Autodesk Fusion 360 part; units mm, degrees
(part 2 of 5)
  spline S63 degree 5 poles (8.5628, 46.3914) (8.5526, 46.3783) (8.5324, 46.3521) (8.5021, 46.3128) (8.4619, 46.2602) (8.4119, 46.1945) (8.3623, 46.1286) (8.3129, 46.0625) (8.2639, 45.9964) (8.2152, 45.9301) (8.1668, 45.8637) (8.1187, 45.7971) (8.0709, 45.7305) (8.0235, 45.6637) (7.9764, 45.5967) (7.9296, 45.5297) (7.8831, 45.4625) (7.837, 45.3952) (7.7912, 45.3278) (7.7458, 45.2602) (7.7007, 45.1925) (7.6639, 45.1368) (7.6362, 45.0946) (7.6175, 45.0659) (7.6077, 45.0508) (7.6067, 45.0493) knots -1 -1 -1 -1 -1 -1 -0.985714 -0.971429 -0.957143 -0.942857 -0.928571 -0.914286 -0.9 -0.885714 -0.871429 -0.857143 -0.842857 -0.828571 -0.814286 -0.8 -0.785714 -0.771429 -0.757143 -0.742857 -0.728571 -0.714286 -0.712736 -0.712736 -0.712736 -0.712736 -0.712736 -0.712736
  line L43 (-7.433, 28.7473) -> (-9.4231, 36.4981)
  line L44 (-10.9838, 27.4883) -> (-13.9296, 34.9285)
  spline S64 degree 5 poles (-12.2983, -44.0007) (-12.2981, -44.0024) (-12.2956, -44.0202) (-12.2909, -44.0541) (-12.2838, -44.1041) (-12.2743, -44.1702) (-12.2623, -44.2506) (-12.2499, -44.3311) (-12.2372, -44.4116) (-12.2241, -44.4922) (-12.2107, -44.5727) (-12.1969, -44.6533) (-12.1828, -44.734) (-12.1683, -44.8146) (-12.1534, -44.8953) (-12.1383, -44.9759) (-12.1228, -45.0566) (-12.1069, -45.1374) (-12.0907, -45.2181) (-12.0742, -45.2989) (-12.0573, -45.3796) (-12.0401, -45.4604) (-12.0261, -45.525) (-12.0154, -45.5735) (-12.0083, -45.6059) (-12.0047, -45.622) knots 0.712736 0.712736 0.712736 0.712736 0.712736 0.712736 0.714286 0.728571 0.742857 0.757143 0.771429 0.785714 0.8 0.814286 0.828571 0.842857 0.857143 0.871429 0.885714 0.9 0.914286 0.928571 0.942857 0.957143 0.971429 0.985714 1 1 1 1 1 1
  arc A63 (-23.9559, 16.8474) -> (-24.9507, 15.2942) centre (0.7975, -0.1016) ccw
  line L45 (22.0846, 21.0374) -> (27.7612, 26.6745)
  line L46 (-21.6364, 19.8162) -> (-27.6188, 25.1276)
  arc A64 (-21.6364, 19.8162) -> (-22.8181, 18.3999) centre (0.7975, -0.1016) ccw
  arc A65 (-37.0211, 3.6065) -> (-37.1692, 1.488) centre (0.7975, -0.1016) ccw
  arc A66 (-9.1163, -46.2858) -> (-8.5628, -46.3914) centre (0, 0) ccw
  spline S65 degree 5 poles (-19.8308, -42.8044) (-19.8177, -42.7943) (-19.7916, -42.7739) (-19.7525, -42.7434) (-19.7005, -42.7025) (-19.6357, -42.6512) (-19.5713, -42.5997) (-19.5071, -42.5481) (-19.4431, -42.4962) (-19.3794, -42.4441) (-19.3161, -42.3918) (-19.2529, -42.3393) (-19.1901, -42.2866) (-19.1275, -42.2337) (-19.0652, -42.1806) (-19.0032, -42.1273) (-18.9415, -42.0738) (-18.8801, -42.02) (-18.819, -41.9661) (-18.7582, -41.912) (-18.6976, -41.8576) (-18.6481, -41.8128) (-18.6109, -41.7788) (-18.5856, -41.7557) (-18.5724, -41.7435) (-18.5711, -41.7423) knots -1 -1 -1 -1 -1 -1 -0.985714 -0.971429 -0.957143 -0.942857 -0.928571 -0.914286 -0.9 -0.885714 -0.871429 -0.857143 -0.842857 -0.828571 -0.814286 -0.8 -0.785714 -0.771429 -0.757143 -0.742857 -0.728571 -0.714286 -0.712736 -0.712736 -0.712736 -0.712736 -0.712736 -0.712736
  spline S66 degree 3 poles (-6.6866, -45.1951) (-6.7038, -45.1309) (-6.7334, -45.0708) (-6.8139, -44.9652) (-6.8641, -44.9207) (-6.9787, -44.8536) (-7.0421, -44.8316) (-7.1736, -44.813) (-7.2405, -44.8167) (-7.3692, -44.8494) (-7.4298, -44.8782) (-7.5318, -44.9539) (-7.5737, -44.9985) (-7.6067, -45.0493) knots 0 0 0 0 0.019923 0.019923 0.039846 0.039846 0.059769 0.059769 0.079691 0.079691 0.099614 0.099614 0.117812 0.117812 0.117812 0.117812
  line L47 (-18.9632, 22.4708) -> (-24.2327, 28.4902)
  line L48 (-29.0593, 2.8259) -> (-37.0211, 3.6065)
  arc A67 (-30.5568, 21.3671) -> (-31.7072, 19.582) centre (0.7975, -0.1016) ccw
  spline S67 degree 3 poles (9.5112, 44.686) (9.5244, 44.621) (9.5501, 44.5591) (9.6239, 44.4486) (9.6712, 44.4011) (9.7814, 44.3269) (9.8432, 44.301) (9.9732, 44.2742) (10.0403, 44.2736) (10.1708, 44.2982) (10.233, 44.3231) (10.3396, 44.3923) (10.3842, 44.4341) (10.4204, 44.4828) knots 0 0 0 0 0.019923 0.019923 0.039846 0.039846 0.059769 0.059769 0.079691 0.079691 0.099614 0.099614 0.117812 0.117812 0.117812 0.117812
  spline S68 degree 3 poles (12.2983, 44.0007) (12.3073, 43.9349) (12.3291, 43.8715) (12.3958, 43.7566) (12.4401, 43.7062) (12.5454, 43.6253) (12.6054, 43.5955) (12.7336, 43.5606) (12.8004, 43.5558) (12.9322, 43.5721) (12.9959, 43.5931) (13.1066, 43.6555) (13.1538, 43.6944) (13.1929, 43.7407) knots 0 0 0 0 0.019923 0.019923 0.039846 0.039846 0.059769 0.059769 0.079691 0.079691 0.099614 0.099614 0.117812 0.117812 0.117812 0.117812
  arc A68 (-25.885, 13.6113) -> (-26.6773, 11.9457) centre (0.7975, -0.1016) ccw
  spline S69 degree 3 poles (6.6866, 45.1951) (6.7038, 45.1309) (6.7334, 45.0708) (6.8139, 44.9652) (6.8641, 44.9207) (6.9787, 44.8536) (7.0421, 44.8316) (7.1736, 44.813) (7.2405, 44.8167) (7.3692, 44.8494) (7.4298, 44.8782) (7.5318, 44.9539) (7.5737, 44.9985) (7.6067, 45.0493) knots 0 0 0 0 0.019923 0.019923 0.039846 0.039846 0.059769 0.059769 0.079691 0.079691 0.099614 0.099614 0.117812 0.117812 0.117812 0.117812
  arc A69 (-12.0047, -45.622) -> (-11.4588, -45.7622) centre (0, 0) ccw
  line L49 (17.7796, 24.6291) -> (22.4832, 31.103)
  arc A70 (-34.9108, 12.8952) -> (-35.5811, 10.88) centre (0.7975, -0.1016) ccw
  line L50 (-24.9507, 15.2942) -> (-31.7072, 19.582)
  spline S70 degree 5 poles (-0.2818, 47.1742) (-0.2893, 47.1594) (-0.3043, 47.1299) (-0.3267, 47.0856) (-0.3563, 47.0264) (-0.3931, 46.9525) (-0.4295, 46.8784) (-0.4656, 46.8043) (-0.5013, 46.7302) (-0.5368, 46.6559) (-0.5719, 46.5816) (-0.6066, 46.5072) (-0.641, 46.4328) (-0.6751, 46.3583) (-0.7089, 46.2837) (-0.7423, 46.2091) (-0.7753, 46.1344) (-0.808, 46.0596) (-0.8404, 45.9848) (-0.8723, 45.9099) (-0.904, 45.835) (-0.9297, 45.7734) (-0.9489, 45.7267) (-0.9619, 45.695) (-0.9687, 45.6784) (-0.9694, 45.6768) knots -1 -1 -1 -1 -1 -1 -0.985714 -0.971429 -0.957143 -0.942857 -0.928571 -0.914286 -0.9 -0.885714 -0.871429 -0.857143 -0.842857 -0.828571 -0.814286 -0.8 -0.785714 -0.771429 -0.757143 -0.742857 -0.728571 -0.714286 -0.712736 -0.712736 -0.712736 -0.712736 -0.712736 -0.712736
  arc A71 (-36.2582, 8.3172) -> (-36.6706, 6.2339) centre (0.7975, -0.1016) ccw
  spline S71 degree 5 poles (19.8308, 42.8044) (19.8177, 42.7943) (19.7916, 42.7739) (19.7525, 42.7434) (19.7005, 42.7025) (19.6357, 42.6512) (19.5713, 42.5997) (19.5071, 42.5481) (19.4431, 42.4962) (19.3794, 42.4441) (19.3161, 42.3918) (19.2529, 42.3393) (19.1901, 42.2866) (19.1275, 42.2337) (19.0652, 42.1806) (19.0032, 42.1273) (18.9415, 42.0738) (18.8801, 42.02) (18.819, 41.9661) (18.7582, 41.912) (18.6976, 41.8576) (18.6481, 41.8128) (18.6109, 41.7788) (18.5856, 41.7557) (18.5724, 41.7435) (18.5711, 41.7423) knots -1 -1 -1 -1 -1 -1 -0.985714 -0.971429 -0.957143 -0.942857 -0.928571 -0.914286 -0.9 -0.885714 -0.871429 -0.857143 -0.842857 -0.828571 -0.814286 -0.8 -0.785714 -0.771429 -0.757143 -0.742857 -0.728571 -0.714286 -0.712736 -0.712736 -0.712736 -0.712736 -0.712736 -0.712736
  spline S72 degree 3 poles (0.9694, 45.6768) (0.9945, 45.6153) (1.0314, 45.5593) (1.1246, 45.4646) (1.1799, 45.4268) (1.3021, 45.3746) (1.3676, 45.3607) (1.5004, 45.3587) (1.5664, 45.3707) (1.69, 45.4194) (1.7465, 45.4555) (1.8382, 45.5434) (1.8742, 45.5929) (1.9006, 45.6475) knots 0 0 0 0 0.019923 0.019923 0.039846 0.039846 0.059769 0.059769 0.079691 0.079691 0.099614 0.099614 0.117812 0.117812 0.117812 0.117812
  spline S73 degree 3 poles (-3.8356, -45.5258) (-3.8568, -45.4628) (-3.8901, -45.4046) (-3.9771, -45.3043) (-4.03, -45.2631) (-4.1486, -45.2033) (-4.2132, -45.1853) (-4.3456, -45.175) (-4.4122, -45.1829) (-4.5386, -45.2236) (-4.5972, -45.2562) (-4.6943, -45.3381) (-4.7333, -45.3852) (-4.7631, -45.4381) knots 0 0 0 0 0.019923 0.019923 0.039846 0.039846 0.059769 0.059769 0.079691 0.079691 0.099614 0.099614 0.117812 0.117812 0.117812 0.117812
  line L51 (-29.1828, 0.9855) -> (-37.1692, 1.488)
  spline S74 degree 5 poles (-5.6329, -46.8375) (-5.6236, -46.8238) (-5.6051, -46.7964) (-5.5773, -46.7552) (-5.5405, -46.7003) (-5.4947, -46.6315) (-5.4493, -46.5626) (-5.4042, -46.4936) (-5.3595, -46.4245) (-5.315, -46.3553) (-5.2709, -46.286) (-5.2271, -46.2165) (-5.1836, -46.147) (-5.1404, -46.0774) (-5.0976, -46.0076) (-5.0551, -45.9377) (-5.013, -45.8678) (-4.9712, -45.7977) (-4.9297, -45.7275) (-4.8886, -45.6572) (-4.8478, -45.5869) (-4.8146, -45.5289) (-4.7896, -45.4851) (-4.7728, -45.4553) (-4.7639, -45.4396) (-4.7631, -45.4381) knots -1 -1 -1 -1 -1 -1 -0.985714 -0.971429 -0.957143 -0.942857 -0.928571 -0.914286 -0.9 -0.885714 -0.871429 -0.857143 -0.842857 -0.828571 -0.814286 -0.8 -0.785714 -0.771429 -0.757143 -0.742857 -0.728571 -0.714286 -0.712736 -0.712736 -0.712736 -0.712736 -0.712736 -0.712736
  spline S75 degree 3 poles (15.0368, 43.1416) (15.0417, 43.0754) (15.0595, 43.0107) (15.1189, 42.8919) (15.1599, 42.8389) (15.2599, 42.7515) (15.3179, 42.718) (15.4436, 42.6751) (15.5101, 42.6661) (15.6426, 42.6741) (15.7075, 42.6911) (15.8219, 42.7464) (15.8714, 42.7823) (15.9134, 42.826) knots 0 0 0 0 0.019923 0.019923 0.039846 0.039846 0.059769 0.059769 0.079691 0.079691 0.099614 0.099614 0.117812 0.117812 0.117812 0.117812
  spline S76 degree 3 poles (-15.0368, -43.1416) (-15.0417, -43.0754) (-15.0595, -43.0107) (-15.1189, -42.8919) (-15.1599, -42.8389) (-15.2599, -42.7515) (-15.3179, -42.718) (-15.4436, -42.6751) (-15.5101, -42.6661) (-15.6426, -42.6741) (-15.7075, -42.6911) (-15.8219, -42.7464) (-15.8714, -42.7823) (-15.9134, -42.826) knots 0 0 0 0 0.019923 0.019923 0.039846 0.039846 0.059769 0.059769 0.079691 0.079691 0.099614 0.099614 0.117812 0.117812 0.117812 0.117812
  spline S77 degree 3 poles (17.7161, 42.1123) (17.7168, 42.0459) (17.7305, 41.9803) (17.7822, 41.858) (17.8198, 41.8024) (17.9141, 41.7089) (17.97, 41.6718) (18.0927, 41.6211) (18.1585, 41.608) (18.2913, 41.6077) (18.3571, 41.6206) (18.4748, 41.6685) (18.5264, 41.7013) (18.5711, 41.7423) knots 0 0 0 0 0.019923 0.019923 0.039846 0.039846 0.059769 0.059769 0.079691 0.079691 0.099614 0.099614 0.117812 0.117812 0.117812 0.117812
  spline S78 degree 5 poles (-17.7161, -42.1123) (-17.716, -42.1141) (-17.7158, -42.1321) (-17.7154, -42.1663) (-17.7147, -42.2168) (-17.7135, -42.2835) (-17.7117, -42.3648) (-17.7095, -42.4462) (-17.707, -42.5277) (-17.7041, -42.6093) (-17.7008, -42.6909) (-17.6973, -42.7726) (-17.6933, -42.8543) (-17.6891, -42.9361) (-17.6845, -43.018) (-17.6795, -43.1) (-17.6743, -43.182) (-17.6686, -43.264) (-17.6627, -43.3462) (-17.6564, -43.4284) (-17.6498, -43.5106) (-17.6429, -43.5929) (-17.6371, -43.6588) (-17.6326, -43.7082) (-17.6295, -43.7412) (-17.628, -43.7577) knots 0.712736 0.712736 0.712736 0.712736 0.712736 0.712736 0.714286 0.728571 0.742857 0.757143 0.771429 0.785714 0.8 0.814286 0.828571 0.842857 0.857143 0.871429 0.885714 0.9 0.914286 0.928571 0.942857 0.957143 0.971429 0.985714 1 1 1 1 1 1
  line L52 (-27.3933, 10.159) -> (-34.9108, 12.8952)
  arc A72 (-1.9215, 29.7749) -> (-3.7524, 29.5514) centre (0.7975, -0.1016) ccw
  spline S79 degree 5 poles (-40.9168, 20.3254) (-40.9186, 20.3254) (-40.9365, 20.3264) (-40.9707, 20.3281) (-41.0211, 20.3305) (-41.0878, 20.3335) (-41.1691, 20.3368) (-41.2505, 20.3398) (-41.332, 20.3423) (-41.4135, 20.3446) (-41.4952, 20.3465) (-41.5769, 20.3481) (-41.6588, 20.3493) (-41.7407, 20.3502) (-41.8227, 20.3507) (-41.9048, 20.3509) (-41.987, 20.3508) (-42.0693, 20.3504) (-42.1516, 20.3496) (-42.234, 20.3485) (-42.3165, 20.347) (-42.3991, 20.3453) (-42.4652, 20.3436) (-42.5148, 20.3422) (-42.5479, 20.3413) (-42.5645, 20.3407) knots 0.712736 0.712736 0.712736 0.712736 0.712736 0.712736 0.714286 0.728571 0.742857 0.757143 0.771429 0.785714 0.8 0.814286 0.828571 0.842857 0.857143 0.871429 0.885714 0.9 0.914286 0.928571 0.942857 0.957143 0.971429 0.985714 1 1 1 1 1 1
  spline S80 degree 5 poles (-45.6768, 0.9694) (-45.6784, 0.9687) (-45.695, 0.9619) (-45.7267, 0.9489) (-45.7734, 0.9297) (-45.835, 0.904) (-45.9099, 0.8723) (-45.9848, 0.8404) (-46.0596, 0.808) (-46.1344, 0.7753) (-46.2091, 0.7423) (-46.2837, 0.7089) (-46.3583, 0.6751) (-46.4328, 0.641) (-46.5072, 0.6066) (-46.5816, 0.5719) (-46.6559, 0.5368) (-46.7302, 0.5013) (-46.8043, 0.4656) (-46.8784, 0.4295) (-46.9525, 0.3931) (-47.0264, 0.3563) (-47.0856, 0.3267) (-47.1299, 0.3043) (-47.1594, 0.2893) (-47.1742, 0.2818) knots 0.712736 0.712736 0.712736 0.712736 0.712736 0.712736 0.714286 0.728571 0.742857 0.757143 0.771429 0.785714 0.8 0.814286 0.828571 0.842857 0.857143 0.871429 0.885714 0.9 0.914286 0.928571 0.942857 0.957143 0.971429 0.985714 1 1 1 1 1 1
  arc A73 (-46.2858, 9.1163) -> (-46.3914, 8.5628) centre (0, 0) ccw
  spline S81 degree 5 poles (-45.1951, 6.6866) (-45.1968, 6.6861) (-45.2142, 6.6815) (-45.2472, 6.6725) (-45.2959, 6.6593) (-45.3603, 6.6415) (-45.4386, 6.6195) (-45.5169, 6.5972) (-45.5952, 6.5744) (-45.6734, 6.5514) (-45.7517, 6.5279) (-45.8299, 6.5042) (-45.9081, 6.48) (-45.9863, 6.4556) (-46.0645, 6.4307) (-46.1426, 6.4056) (-46.2207, 6.3801) (-46.2988, 6.3542) (-46.3769, 6.328) (-46.455, 6.3015) (-46.533, 6.2747) (-46.611, 6.2475) (-46.6733, 6.2255) (-46.7201, 6.2088) (-46.7513, 6.1976) (-46.7669, 6.192) knots 0.712736 0.712736 0.712736 0.712736 0.712736 0.712736 0.714286 0.728571 0.742857 0.757143 0.771429 0.785714 0.8 0.814286 0.828571 0.842857 0.857143 0.871429 0.885714 0.9 0.914286 0.928571 0.942857 0.957143 0.971429 0.985714 1 1 1 1 1 1
  arc A74 (-7.3624, 37.0119) -> (-9.4231, 36.4981) centre (0.7975, -0.1016) ccw
  spline S82 degree 3 poles (-44.686, 9.5112) (-44.621, 9.5244) (-44.5591, 9.5501) (-44.4486, 9.6239) (-44.4011, 9.6712) (-44.3269, 9.7814) (-44.301, 9.8432) (-44.2742, 9.9732) (-44.2736, 10.0403) (-44.2982, 10.1708) (-44.3231, 10.233) (-44.3923, 10.3396) (-44.4341, 10.3842) (-44.4828, 10.4204) knots 0 0 0 0 0.019923 0.019923 0.039846 0.039846 0.059769 0.059769 0.079691 0.079691 0.099614 0.099614 0.117812 0.117812 0.117812 0.117812
  spline S83 degree 5 poles (-9.1163, 46.2858) (-9.121, 46.2699) (-9.1301, 46.2381) (-9.1438, 46.1903) (-9.1619, 46.1267) (-9.1841, 46.0472) (-9.206, 45.9676) (-9.2276, 45.8881) (-9.2488, 45.8085) (-9.2697, 45.7289) (-9.2903, 45.6494) (-9.3105, 45.5698) (-9.3303, 45.4902) (-9.3498, 45.4106) (-9.369, 45.3311) (-9.3878, 45.2515) (-9.4063, 45.1719) (-9.4244, 45.0924) (-9.4422, 45.0128) (-9.4596, 44.9333) (-9.4766, 44.8537) (-9.4903, 44.7884) (-9.5005, 44.7389) (-9.5073, 44.7054) (-9.5109, 44.6878) (-9.5112, 44.686) knots -1 -1 -1 -1 -1 -1 -0.985714 -0.971429 -0.957143 -0.942857 -0.928571 -0.914286 -0.9 -0.885714 -0.871429 -0.857143 -0.842857 -0.828571 -0.814286 -0.8 -0.785714 -0.771429 -0.757143 -0.742857 -0.728571 -0.714286 -0.712736 -0.712736 -0.712736 -0.712736 -0.712736 -0.712736
  arc A75 (14.8456, 44.7782) -> (14.3096, 44.9524) centre (0, 0) ccw
  spline S84 degree 5 poles (-46.3914, 8.5628) (-46.3783, 8.5526) (-46.3521, 8.5324) (-46.3128, 8.5021) (-46.2602, 8.4619) (-46.1945, 8.4119) (-46.1286, 8.3623) (-46.0625, 8.3129) (-45.9964, 8.2639) (-45.9301, 8.2152) (-45.8637, 8.1668) (-45.7971, 8.1187) (-45.7305, 8.0709) (-45.6637, 8.0235) (-45.5967, 7.9764) (-45.5297, 7.9296) (-45.4625, 7.8831) (-45.3952, 7.837) (-45.3278, 7.7912) (-45.2602, 7.7458) (-45.1925, 7.7007) (-45.1368, 7.6639) (-45.0946, 7.6362) (-45.0659, 7.6175) (-45.0508, 7.6077) (-45.0493, 7.6067) knots -1 -1 -1 -1 -1 -1 -0.985714 -0.971429 -0.957143 -0.942857 -0.928571 -0.914286 -0.9 -0.885714 -0.871429 -0.857143 -0.842857 -0.828571 -0.814286 -0.8 -0.785714 -0.771429 -0.757143 -0.742857 -0.728571 -0.714286 -0.712736 -0.712736 -0.712736 -0.712736 -0.712736 -0.712736
  arc A76 (-16.3358, 33.8167) -> (-18.204, 32.8065) centre (0.7975, -0.1016) ccw
  line L53 (-1.9215, 29.7749) -> (-2.6465, 37.742)
  spline S85 degree 5 poles (11.4588, 45.7622) (11.4479, 45.7497) (11.426, 45.7249) (11.3933, 45.6875) (11.3499, 45.6376) (11.2959, 45.5751) (11.2422, 45.5125) (11.1888, 45.4497) (11.1357, 45.3867) (11.083, 45.3236) (11.0305, 45.2604) (10.9783, 45.197) (10.9265, 45.1334) (10.8749, 45.0698) (10.8237, 45.0059) (10.7728, 44.9419) (10.7222, 44.8778) (10.6719, 44.8135) (10.622, 44.7491) (10.5724, 44.6845) (10.5231, 44.6198) (10.4829, 44.5665) (10.4526, 44.5261) (10.4322, 44.4987) (10.4215, 44.4842) (10.4204, 44.4828) knots -1 -1 -1 -1 -1 -1 -0.985714 -0.971429 -0.957143 -0.942857 -0.928571 -0.914286 -0.9 -0.885714 -0.871429 -0.857143 -0.842857 -0.828571 -0.814286 -0.8 -0.785714 -0.771429 -0.757143 -0.742857 -0.728571 -0.714286 -0.712736 -0.712736 -0.712736 -0.712736 -0.712736 -0.712736
  spline S86 degree 3 poles (-18.5711, 41.7423) (-18.5222, 41.6974) (-18.465, 41.6624) (-18.3404, 41.6164) (-18.2742, 41.6058) (-18.1414, 41.6106) (-18.0762, 41.6259) (-17.9552, 41.6807) (-17.9006, 41.7196) (-17.8095, 41.8162) (-17.7738, 41.873) (-17.7282, 41.9916) (-17.7167, 42.0517) (-17.7161, 42.1123) knots 0 0 0 0 0.019923 0.019923 0.039846 0.039846 0.059769 0.059769 0.079691 0.079691 0.099614 0.099614 0.117812 0.117812 0.117812 0.117812
  spline S87 degree 5 poles (6.6866, 45.1951) (6.6861, 45.1968) (6.6815, 45.2142) (6.6725, 45.2472) (6.6593, 45.2959) (6.6415, 45.3603) (6.6195, 45.4386) (6.5972, 45.5169) (6.5744, 45.5952) (6.5514, 45.6734) (6.5279, 45.7517) (6.5042, 45.8299) (6.48, 45.9081) (6.4556, 45.9863) (6.4307, 46.0645) (6.4056, 46.1426) (6.3801, 46.2207) (6.3542, 46.2988) (6.328, 46.3769) (6.3015, 46.455) (6.2747, 46.533) (6.2475, 46.611) (6.2255, 46.6733) (6.2088, 46.7201) (6.1976, 46.7513) (6.192, 46.7669) knots 0.712736 0.712736 0.712736 0.712736 0.712736 0.712736 0.714286 0.728571 0.742857 0.757143 0.771429 0.785714 0.8 0.814286 0.828571 0.842857 0.857143 0.871429 0.885714 0.9 0.914286 0.928571 0.942857 0.957143 0.971429 0.985714 1 1 1 1 1 1
  spline S88 degree 3 poles (-44.0007, 12.2983) (-43.9349, 12.3073) (-43.8715, 12.3291) (-43.7566, 12.3958) (-43.7062, 12.4401) (-43.6253, 12.5454) (-43.5955, 12.6054) (-43.5606, 12.7336) (-43.5558, 12.8004) (-43.5721, 12.9322) (-43.5931, 12.9959) (-43.6555, 13.1066) (-43.6944, 13.1538) (-43.7407, 13.1929) knots 0 0 0 0 0.019923 0.019923 0.039846 0.039846 0.059769 0.059769 0.079691 0.079691 0.099614 0.099614 0.117812 0.117812 0.117812 0.117812
  arc A77 (-20.3407, -42.5645) -> (-19.8308, -42.8044) centre (0, 0) ccw
  arc A78 (-5.6329, 46.8375) -> (-6.192, 46.7669) centre (0, 0) ccw
  line L54 (-12.7288, 26.676) -> (-16.3358, 33.8167)
  spline S89 degree 5 poles (17.7161, 42.1123) (17.716, 42.1141) (17.7158, 42.1321) (17.7154, 42.1663) (17.7147, 42.2168) (17.7135, 42.2835) (17.7117, 42.3648) (17.7095, 42.4462) (17.707, 42.5277) (17.7041, 42.6093) (17.7008, 42.6909) (17.6973, 42.7726) (17.6933, 42.8543) (17.6891, 42.9361) (17.6845, 43.018) (17.6795, 43.1) (17.6743, 43.182) (17.6686, 43.264) (17.6627, 43.3462) (17.6564, 43.4284) (17.6498, 43.5106) (17.6429, 43.5929) (17.6371, 43.6588) (17.6326, 43.7082) (17.6295, 43.7412) (17.628, 43.7577) knots 0.712736 0.712736 0.712736 0.712736 0.712736 0.712736 0.714286 0.728571 0.742857 0.757143 0.771429 0.785714 0.8 0.814286 0.828571 0.842857 0.857143 0.871429 0.885714 0.9 0.914286 0.928571 0.942857 0.957143 0.971429 0.985714 1 1 1 1 1 1
  spline S90 degree 5 poles (-9.5112, -44.686) (-9.5109, -44.6878) (-9.5073, -44.7054) (-9.5005, -44.7389) (-9.4903, -44.7884) (-9.4766, -44.8537) (-9.4596, -44.9333) (-9.4422, -45.0128) (-9.4244, -45.0924) (-9.4063, -45.1719) (-9.3878, -45.2515) (-9.369, -45.3311) (-9.3498, -45.4106) (-9.3303, -45.4902) (-9.3105, -45.5698) (-9.2903, -45.6494) (-9.2697, -45.7289) (-9.2488, -45.8085) (-9.2276, -45.8881) (-9.206, -45.9676) (-9.1841, -46.0472) (-9.1619, -46.1267) (-9.1438, -46.1903) (-9.1301, -46.2381) (-9.121, -46.2699) (-9.1163, -46.2858) knots 0.712736 0.712736 0.712736 0.712736 0.712736 0.712736 0.714286 0.728571 0.742857 0.757143 0.771429 0.785714 0.8 0.814286 0.828571 0.842857 0.857143 0.871429 0.885714 0.9 0.914286 0.928571 0.942857 0.957143 0.971429 0.985714 1 1 1 1 1 1
  spline S91 degree 5 poles (9.5112, 44.686) (9.5109, 44.6878) (9.5073, 44.7054) (9.5005, 44.7389) (9.4903, 44.7884) (9.4766, 44.8537) (9.4596, 44.9333) (9.4422, 45.0128) (9.4244, 45.0924) (9.4063, 45.1719) (9.3878, 45.2515) (9.369, 45.3311) (9.3498, 45.4106) (9.3303, 45.4902) (9.3105, 45.5698) (9.2903, 45.6494) (9.2697, 45.7289) (9.2488, 45.8085) (9.2276, 45.8881) (9.206, 45.9676) (9.1841, 46.0472) (9.1619, 46.1267) (9.1438, 46.1903) (9.1301, 46.2381) (9.121, 46.2699) (9.1163, 46.2858) knots 0.712736 0.712736 0.712736 0.712736 0.712736 0.712736 0.714286 0.728571 0.742857 0.757143 0.771429 0.785714 0.8 0.814286 0.828571 0.842857 0.857143 0.871429 0.885714 0.9 0.914286 0.928571 0.942857 0.957143 0.971429 0.985714 1 1 1 1 1 1
  arc A79 (-2.6465, 37.742) -> (-4.7553, 37.4905) centre (0.7975, -0.1016) ccw
  arc A80 (-22.9733, -41.2033) -> (-22.4794, -41.4748) centre (0, 0) ccw
  spline S92 degree 3 poles (-25.2933, -38.0467) (-25.2816, -37.9814) (-25.2827, -37.9143) (-25.3107, -37.7845) (-25.3372, -37.7229) (-25.4123, -37.6134) (-25.4602, -37.5665) (-25.5713, -37.4937) (-25.6334, -37.4685) (-25.7638, -37.4433) (-25.8309, -37.4436) (-25.9554, -37.4686) (-26.0123, -37.4911) (-26.0639, -37.5231) knots 0 0 0 0 0.019923 0.019923 0.039846 0.039846 0.059769 0.059769 0.079691 0.079691 0.099614 0.099614 0.117812 0.117812 0.117812 0.117812
  spline S93 degree 5 poles (-43.9652, 17.104) (-43.9542, 17.0916) (-43.9323, 17.0668) (-43.8993, 17.0296) (-43.8553, 16.9803) (-43.8, 16.9189) (-43.7446, 16.8578) (-43.689, 16.7969) (-43.6332, 16.7364) (-43.5772, 16.6761) (-43.521, 16.6161) (-43.4646, 16.5564) (-43.4081, 16.497) (-43.3514, 16.4379) (-43.2945, 16.3791) (-43.2374, 16.3206) (-43.1801, 16.2623) (-43.1226, 16.2044) (-43.065, 16.1468) (-43.0071, 16.0895) (-42.9491, 16.0325) (-42.9012, 15.9859) (-42.8649, 15.9508) (-42.8403, 15.9271) (-42.8273, 15.9146) (-42.826, 15.9134) knots -1 -1 -1 -1 -1 -1 -0.985714 -0.971429 -0.957143 -0.942857 -0.928571 -0.914286 -0.9 -0.885714 -0.871429 -0.857143 -0.842857 -0.828571 -0.814286 -0.8 -0.785714 -0.771429 -0.757143 -0.742857 -0.728571 -0.714286 -0.712736 -0.712736 -0.712736 -0.712736 -0.712736 -0.712736
  spline S94 degree 5 poles (0.9694, 45.6768) (0.9687, 45.6784) (0.9619, 45.695) (0.9489, 45.7267) (0.9297, 45.7734) (0.904, 45.835) (0.8723, 45.9099) (0.8404, 45.9848) (0.808, 46.0596) (0.7753, 46.1344) (0.7423, 46.2091) (0.7089, 46.2837) (0.6751, 46.3583) (0.641, 46.4328) (0.6066, 46.5072) (0.5719, 46.5816) (0.5368, 46.6559) (0.5013, 46.7302) (0.4656, 46.8043) (0.4295, 46.8784) (0.3931, 46.9525) (0.3563, 47.0264) (0.3267, 47.0856) (0.3043, 47.1299) (0.2893, 47.1594) (0.2818, 47.1742) knots 0.712736 0.712736 0.712736 0.712736 0.712736 0.712736 0.714286 0.728571 0.742857 0.757143 0.771429 0.785714 0.8 0.814286 0.828571 0.842857 0.857143 0.871429 0.885714 0.9 0.914286 0.928571 0.942857 0.957143 0.971429 0.985714 1 1 1 1 1 1
  spline S95 degree 3 poles (-45.1951, 6.6866) (-45.1309, 6.7038) (-45.0708, 6.7334) (-44.9652, 6.8139) (-44.9207, 6.8641) (-44.8536, 6.9787) (-44.8316, 7.0421) (-44.813, 7.1736) (-44.8167, 7.2405) (-44.8494, 7.3692) (-44.8782, 7.4298) (-44.9539, 7.5318) (-44.9985, 7.5737) (-45.0493, 7.6067) knots 0 0 0 0 0.019923 0.019923 0.039846 0.039846 0.059769 0.059769 0.079691 0.079691 0.099614 0.099614 0.117812 0.117812 0.117812 0.117812
  spline S96 degree 5 poles (17.104, 43.9652) (17.0916, 43.9542) (17.0668, 43.9323) (17.0296, 43.8993) (16.9803, 43.8553) (16.9189, 43.8) (16.8578, 43.7446) (16.7969, 43.689) (16.7364, 43.6332) (16.6761, 43.5772) (16.6161, 43.521) (16.5564, 43.4646) (16.497, 43.4081) (16.4379, 43.3514) (16.3791, 43.2945) (16.3206, 43.2374) (16.2623, 43.1801) (16.2044, 43.1226) (16.1468, 43.065) (16.0895, 43.0071) (16.0325, 42.9491) (15.9859, 42.9012) (15.9508, 42.8649) (15.9271, 42.8403) (15.9146, 42.8273) (15.9134, 42.826) knots -1 -1 -1 -1 -1 -1 -0.985714 -0.971429 -0.957143 -0.942857 -0.928571 -0.914286 -0.9 -0.885714 -0.871429 -0.857143 -0.842857 -0.828571 -0.814286 -0.8 -0.785714 -0.771429 -0.757143 -0.742857 -0.728571 -0.714286 -0.712736 -0.712736 -0.712736 -0.712736 -0.712736 -0.712736
  spline S97 degree 5 poles (-41.4748, 22.4794) (-41.4655, 22.4657) (-41.4468, 22.4383) (-41.4188, 22.3974) (-41.3812, 22.3429) (-41.3341, 22.2751) (-41.2868, 22.2075) (-41.2392, 22.1402) (-41.1915, 22.0731) (-41.1435, 22.0063) (-41.0953, 21.9397) (-41.0468, 21.8734) (-40.9982, 21.8074) (-40.9493, 21.7417) (-40.9002, 21.6762) (-40.8509, 21.6109) (-40.8014, 21.546) (-40.7516, 21.4813) (-40.7016, 21.4169) (-40.6514, 21.3528) (-40.601, 21.289) (-40.5594, 21.2368) (-40.5278, 21.1974) (-40.5063, 21.1708) (-40.495, 21.1568) (-40.4939, 21.1555) knots -1 -1 -1 -1 -1 -1 -0.985714 -0.971429 -0.957143 -0.942857 -0.928571 -0.914286 -0.9 -0.885714 -0.871429 -0.857143 -0.842857 -0.828571 -0.814286 -0.8 -0.785714 -0.771429 -0.757143 -0.742857 -0.728571 -0.714286 -0.712736 -0.712736 -0.712736 -0.712736 -0.712736 -0.712736
  arc A81 (12.0047, 45.622) -> (11.4588, 45.7622) centre (0, 0) ccw
  spline S98 degree 5 poles (-8.5628, -46.3914) (-8.5526, -46.3783) (-8.5324, -46.3521) (-8.5021, -46.3128) (-8.4619, -46.2602) (-8.4119, -46.1945) (-8.3623, -46.1286) (-8.3129, -46.0625) (-8.2639, -45.9964) (-8.2152, -45.9301) (-8.1668, -45.8637) (-8.1187, -45.7971) (-8.0709, -45.7305) (-8.0235, -45.6637) (-7.9764, -45.5967) (-7.9296, -45.5297) (-7.8831, -45.4625) (-7.837, -45.3952) (-7.7912, -45.3278) (-7.7458, -45.2602) (-7.7007, -45.1925) (-7.6639, -45.1368) (-7.6362, -45.0946) (-7.6175, -45.0659) (-7.6077, -45.0508) (-7.6067, -45.0493) knots -1 -1 -1 -1 -1 -1 -0.985714 -0.971429 -0.957143 -0.942857 -0.928571 -0.914286 -0.9 -0.885714 -0.871429 -0.857143 -0.842857 -0.828571 -0.814286 -0.8 -0.785714 -0.771429 -0.757143 -0.742857 -0.728571 -0.714286 -0.712736 -0.712736 -0.712736 -0.712736 -0.712736 -0.712736
  spline S99 degree 5 poles (3.8356, 45.5258) (3.835, 45.5274) (3.8292, 45.5445) (3.8183, 45.5769) (3.802, 45.6247) (3.7802, 45.6878) (3.7533, 45.7646) (3.7261, 45.8413) (3.6985, 45.918) (3.6706, 45.9947) (3.6423, 46.0713) (3.6137, 46.1479) (3.5847, 46.2244) (3.5553, 46.3009) (3.5256, 46.3774) (3.4956, 46.4538) (3.4653, 46.5301) (3.4346, 46.6065) (3.4035, 46.6827) (3.3722, 46.759) (3.3405, 46.8351) (3.3084, 46.9113) (3.2825, 46.9721) (3.263, 47.0178) (3.2499, 47.0482) (3.2433, 47.0634) knots 0.712736 0.712736 0.712736 0.712736 0.712736 0.712736 0.714286 0.728571 0.742857 0.757143 0.771429 0.785714 0.8 0.814286 0.828571 0.842857 0.857143 0.871429 0.885714 0.9 0.914286 0.928571 0.942857 0.957143 0.971429 0.985714 1 1 1 1 1 1
  spline S100 degree 3 poles (-43.1416, 15.0368) (-43.0754, 15.0417) (-43.0107, 15.0595) (-42.8919, 15.1189) (-42.8389, 15.1599) (-42.7515, 15.2599) (-42.718, 15.3179) (-42.6751, 15.4436) (-42.6661, 15.5101) (-42.6741, 15.6426) (-42.6911, 15.7075) (-42.7464, 15.8219) (-42.7823, 15.8714) (-42.826, 15.9134) knots 0 0 0 0 0.019923 0.019923 0.039846 0.039846 0.059769 0.059769 0.079691 0.079691 0.099614 0.099614 0.117812 0.117812 0.117812 0.117812
  spline S101 degree 3 poles (20.3254, 40.9168) (20.3219, 40.8505) (20.3314, 40.7841) (20.3754, 40.6588) (20.4094, 40.601) (20.4977, 40.5018) (20.5511, 40.4613) (20.6705, 40.403) (20.7352, 40.3857) (20.8678, 40.3771) (20.9343, 40.3858) (21.0547, 40.4263) (21.1083, 40.4557) (21.1555, 40.4939) knots 0 0 0 0 0.019923 0.019923 0.039846 0.039846 0.059769 0.059769 0.079691 0.079691 0.099614 0.099614 0.117812 0.117812 0.117812 0.117812
  spline S102 degree 5 poles (-43.1416, 15.0368) (-43.1434, 15.0367) (-43.1613, 15.0354) (-43.1954, 15.0328) (-43.2458, 15.0289) (-43.3123, 15.0235) (-43.3934, 15.0166) (-43.4745, 15.0093) (-43.5556, 15.0017) (-43.6368, 14.9937) (-43.7181, 14.9853) (-43.7994, 14.9766) (-43.8807, 14.9676) (-43.9621, 14.9582) (-44.0436, 14.9485) (-44.125, 14.9384) (-44.2065, 14.928) (-44.2881, 14.9172) (-44.3697, 14.9061) (-44.4513, 14.8947) (-44.533, 14.8829) (-44.6147, 14.8709) (-44.6801, 14.8609) (-44.7291, 14.8533) (-44.7619, 14.8482) (-44.7782, 14.8456) knots 0.712736 0.712736 0.712736 0.712736 0.712736 0.712736 0.714286 0.728571 0.742857 0.757143 0.771429 0.785714 0.8 0.814286 0.828571 0.842857 0.857143 0.871429 0.885714 0.9 0.914286 0.928571 0.942857 0.957143 0.971429 0.985714 1 1 1 1 1 1
  arc A82 (17.628, 43.7577) -> (17.104, 43.9652) centre (0, 0) ccw
  spline S103 degree 3 poles (-7.6067, 45.0493) (-7.5705, 44.9937) (-7.5238, 44.9456) (-7.4146, 44.87) (-7.3531, 44.8433) (-7.2234, 44.8149) (-7.1563, 44.8135) (-7.0255, 44.8365) (-6.963, 44.8606) (-6.8507, 44.9315) (-6.802, 44.9776) (-6.7283, 45.0812) (-6.7023, 45.1365) (-6.6866, 45.1951) knots 0 0 0 0 0.019923 0.019923 0.039846 0.039846 0.059769 0.059769 0.079691 0.079691 0.099614 0.099614 0.117812 0.117812 0.117812 0.117812
  spline S104 degree 5 poles (27.6324, 36.3835) (27.6328, 36.3852) (27.6371, 36.4027) (27.6452, 36.4359) (27.657, 36.485) (27.6725, 36.5499) (27.6909, 36.6292) (27.7091, 36.7085) (27.7269, 36.7881) (27.7444, 36.8678) (27.7615, 36.9476) (27.7784, 37.0277) (27.7949, 37.1078) (27.8111, 37.1881) (27.827, 37.2686) (27.8426, 37.3492) (27.8579, 37.4299) (27.8729, 37.5108) (27.8875, 37.5918) (27.9019, 37.673) (27.916, 37.7543) (27.9297, 37.8358) (27.9405, 37.901) (27.9484, 37.95) (27.9536, 37.9827) (27.9562, 37.9991) knots 0.712736 0.712736 0.712736 0.712736 0.712736 0.712736 0.714286 0.728571 0.742857 0.757143 0.771429 0.785714 0.8 0.814286 0.828571 0.842857 0.857143 0.871429 0.885714 0.9 0.914286 0.928571 0.942857 0.957143 0.971429 0.985714 1 1 1 1 1 1
  spline S105 degree 3 poles (-17.7161, -42.1123) (-17.7168, -42.0459) (-17.7305, -41.9803) (-17.7822, -41.858) (-17.8198, -41.8024) (-17.9141, -41.7089) (-17.97, -41.6718) (-18.0927, -41.6211) (-18.1585, -41.608) (-18.2913, -41.6077) (-18.3571, -41.6206) (-18.4748, -41.6685) (-18.5264, -41.7013) (-18.5711, -41.7423) knots 0 0 0 0 0.019923 0.019923 0.039846 0.039846 0.059769 0.059769 0.079691 0.079691 0.099614 0.099614 0.117812 0.117812 0.117812 0.117812
  spline S106 degree 3 poles (-45.5258, 3.8356) (-45.4628, 3.8568) (-45.4046, 3.8901) (-45.3043, 3.9771) (-45.2631, 4.03) (-45.2033, 4.1486) (-45.1853, 4.2132) (-45.175, 4.3456) (-45.1829, 4.4122) (-45.2236, 4.5386) (-45.2562, 4.5972) (-45.3381, 4.6943) (-45.3852, 4.7333) (-45.4381, 4.7631) knots 0 0 0 0 0.019923 0.019923 0.039846 0.039846 0.059769 0.059769 0.079691 0.079691 0.099614 0.099614 0.117812 0.117812 0.117812 0.117812
  spline S107 degree 3 poles (-4.7631, 45.4381) (-4.7304, 45.3802) (-4.6868, 45.3293) (-4.5825, 45.2471) (-4.5229, 45.2165) (-4.3952, 45.18) (-4.3283, 45.1744) (-4.1963, 45.1891) (-4.1324, 45.2093) (-4.0159, 45.273) (-3.9644, 45.316) (-3.8844, 45.4147) (-3.8549, 45.4683) (-3.8356, 45.5258) knots 0 0 0 0 0.019923 0.019923 0.039846 0.039846 0.059769 0.059769 0.079691 0.079691 0.099614 0.099614 0.117812 0.117812 0.117812 0.117812
  spline S108 degree 3 poles (-40.9168, 20.3254) (-40.8505, 20.3219) (-40.7841, 20.3314) (-40.6588, 20.3754) (-40.601, 20.4094) (-40.5018, 20.4977) (-40.4613, 20.5511) (-40.403, 20.6705) (-40.3857, 20.7352) (-40.3771, 20.8678) (-40.3858, 20.9343) (-40.4263, 21.0547) (-40.4557, 21.1083) (-40.4939, 21.1555) knots 0 0 0 0 0.019923 0.019923 0.039846 0.039846 0.059769 0.059769 0.079691 0.079691 0.099614 0.099614 0.117812 0.117812 0.117812 0.117812
  spline S109 degree 5 poles (-27.6324, -36.3835) (-27.6328, -36.3852) (-27.6371, -36.4027) (-27.6452, -36.4359) (-27.657, -36.485) (-27.6725, -36.5499) (-27.6909, -36.6292) (-27.7091, -36.7085) (-27.7269, -36.7881) (-27.7444, -36.8678) (-27.7615, -36.9476) (-27.7784, -37.0277) (-27.7949, -37.1078) (-27.8111, -37.1881) (-27.827, -37.2686) (-27.8426, -37.3492) (-27.8579, -37.4299) (-27.8729, -37.5108) (-27.8875, -37.5918) (-27.9019, -37.673) (-27.916, -37.7543) (-27.9297, -37.8358) (-27.9405, -37.901) (-27.9484, -37.95) (-27.9536, -37.9827) (-27.9562, -37.9991) knots 0.712736 0.712736 0.712736 0.712736 0.712736 0.712736 0.714286 0.728571 0.742857 0.757143 0.771429 0.785714 0.8 0.814286 0.828571 0.842857 0.857143 0.871429 0.885714 0.9 0.914286 0.928571 0.942857 0.957143 0.971429 0.985714 1 1 1 1 1 1
  arc A83 (-12.7288, 26.676) -> (-14.3489, 25.7941) centre (0.7975, -0.1016) ccw
  arc A84 (9.1163, 46.2858) -> (8.5628, 46.3914) centre (0, 0) ccw
  spline S110 degree 5 poles (12.2983, 44.0007) (12.2981, 44.0024) (12.2956, 44.0202) (12.2909, 44.0541) (12.2838, 44.1041) (12.2743, 44.1702) (12.2623, 44.2506) (12.2499, 44.3311) (12.2372, 44.4116) (12.2241, 44.4922) (12.2107, 44.5727) (12.1969, 44.6533) (12.1828, 44.734) (12.1683, 44.8146) (12.1534, 44.8953) (12.1383, 44.9759) (12.1228, 45.0566) (12.1069, 45.1374) (12.0907, 45.2181) (12.0742, 45.2989) (12.0573, 45.3796) (12.0401, 45.4604) (12.0261, 45.525) (12.0154, 45.5735) (12.0083, 45.6059) (12.0047, 45.622) knots 0.712736 0.712736 0.712736 0.712736 0.712736 0.712736 0.714286 0.728571 0.742857 0.757143 0.771429 0.785714 0.8 0.814286 0.828571 0.842857 0.857143 0.871429 0.885714 0.9 0.914286 0.928571 0.942857 0.957143 0.971429 0.985714 1 1 1 1 1 1
  spline S111 degree 5 poles (-20.3254, -40.9168) (-20.3254, -40.9186) (-20.3264, -40.9365) (-20.3281, -40.9707) (-20.3305, -41.0211) (-20.3335, -41.0878) (-20.3368, -41.1691) (-20.3398, -41.2505) (-20.3423, -41.332) (-20.3446, -41.4135) (-20.3465, -41.4952) (-20.3481, -41.5769) (-20.3493, -41.6588) (-20.3502, -41.7407) (-20.3507, -41.8227) (-20.3509, -41.9048) (-20.3508, -41.987) (-20.3504, -42.0693) (-20.3496, -42.1516) (-20.3485, -42.234) (-20.347, -42.3165) (-20.3453, -42.3991) (-20.3436, -42.4652) (-20.3422, -42.5148) (-20.3413, -42.5479) (-20.3407, -42.5645) knots 0.712736 0.712736 0.712736 0.712736 0.712736 0.712736 0.714286 0.728571 0.742857 0.757143 0.771429 0.785714 0.8 0.814286 0.828571 0.842857 0.857143 0.871429 0.885714 0.9 0.914286 0.928571 0.942857 0.957143 0.971429 0.985714 1 1 1 1 1 1
  spline S112 degree 5 poles (2.6809, 47.0988) (2.6724, 47.0845) (2.6556, 47.056) (2.6305, 47.0132) (2.5972, 46.956) (2.5559, 46.8845) (2.5149, 46.8129) (2.4742, 46.7412) (2.4339, 46.6694) (2.3938, 46.5976) (2.3542, 46.5256) (2.3148, 46.4536) (2.2758, 46.3814) (2.2371, 46.3092) (2.1987, 46.2369) (2.1607, 46.1645) (2.123, 46.092) (2.0857, 46.0195) (2.0487, 45.9468) (2.0121, 45.8741) (1.9758, 45.8013) (1.9463, 45.7414) (1.9241, 45.6961) (1.9092, 45.6653) (1.9013, 45.6491) (1.9006, 45.6475) knots -1 -1 -1 -1 -1 -1 -0.985714 -0.971429 -0.957143 -0.942857 -0.928571 -0.914286 -0.9 -0.885714 -0.871429 -0.857143 -0.842857 -0.828571 -0.814286 -0.8 -0.785714 -0.771429 -0.757143 -0.742857 -0.728571 -0.714286 -0.712736 -0.712736 -0.712736 -0.712736 -0.712736 -0.712736
  arc A85 (-9.266, 28.1601) -> (-10.9838, 27.4883) centre (0.7975, -0.1016) ccw
  spline S113 degree 5 poles (-17.104, -43.9652) (-17.0916, -43.9542) (-17.0668, -43.9323) (-17.0296, -43.8993) (-16.9803, -43.8553) (-16.9189, -43.8) (-16.8578, -43.7446) (-16.7969, -43.689) (-16.7364, -43.6332) (-16.6761, -43.5772) (-16.6161, -43.521) (-16.5564, -43.4646) (-16.497, -43.4081) (-16.4379, -43.3514) (-16.3791, -43.2945) (-16.3206, -43.2374) (-16.2623, -43.1801) (-16.2044, -43.1226) (-16.1468, -43.065) (-16.0895, -43.0071) (-16.0325, -42.9491) (-15.9859, -42.9012) (-15.9508, -42.8649) (-15.9271, -42.8403) (-15.9146, -42.8273) (-15.9134, -42.826) knots -1 -1 -1 -1 -1 -1 -0.985714 -0.971429 -0.957143 -0.942857 -0.928571 -0.914286 -0.9 -0.885714 -0.871429 -0.857143 -0.842857 -0.828571 -0.814286 -0.8 -0.785714 -0.771429 -0.757143 -0.742857 -0.728571 -0.714286 -0.712736 -0.712736 -0.712736 -0.712736 -0.712736 -0.712736
  arc A86 (-17.628, -43.7577) -> (-17.104, -43.9652) centre (0, 0) ccw
  spline S114 degree 5 poles (15.0368, 43.1416) (15.0367, 43.1434) (15.0354, 43.1613) (15.0328, 43.1954) (15.0289, 43.2458) (15.0235, 43.3123) (15.0166, 43.3934) (15.0093, 43.4745) (15.0017, 43.5556) (14.9937, 43.6368) (14.9853, 43.7181) (14.9766, 43.7994) (14.9676, 43.8807) (14.9582, 43.9621) (14.9485, 44.0436) (14.9384, 44.125) (14.928, 44.2065) (14.9172, 44.2881) (14.9061, 44.3697) (14.8947, 44.4513) (14.8829, 44.533) (14.8709, 44.6147) (14.8609, 44.6801) (14.8533, 44.7291) (14.8482, 44.7619) (14.8456, 44.7782) knots 0.712736 0.712736 0.712736 0.712736 0.712736 0.712736 0.714286 0.728571 0.742857 0.757143 0.771429 0.785714 0.8 0.814286 0.828571 0.842857 0.857143 0.871429 0.885714 0.9 0.914286 0.928571 0.942857 0.957143 0.971429 0.985714 1 1 1 1 1 1
  spline S115 degree 5 poles (-6.6866, -45.1951) (-6.6861, -45.1968) (-6.6815, -45.2142) (-6.6725, -45.2472) (-6.6593, -45.2959) (-6.6415, -45.3603) (-6.6195, -45.4386) (-6.5972, -45.5169) (-6.5744, -45.5952) (-6.5514, -45.6734) (-6.5279, -45.7517) (-6.5042, -45.8299) (-6.48, -45.9081) (-6.4556, -45.9863) (-6.4307, -46.0645) (-6.4056, -46.1426) (-6.3801, -46.2207) (-6.3542, -46.2988) (-6.328, -46.3769) (-6.3015, -46.455) (-6.2747, -46.533) (-6.2475, -46.611) (-6.2255, -46.6733) (-6.2088, -46.7201) (-6.1976, -46.7513) (-6.192, -46.7669) knots 0.712736 0.712736 0.712736 0.712736 0.712736 0.712736 0.714286 0.728571 0.742857 0.757143 0.771429 0.785714 0.8 0.814286 0.828571 0.842857 0.857143 0.871429 0.885714 0.9 0.914286 0.928571 0.942857 0.957143 0.971429 0.985714 1 1 1 1 1 1
  arc A87 (-11.9496, 35.6966) -> (-13.9296, 34.9285) centre (0.7975, -0.1016) ccw
  spline S116 degree 5 poles (-15.0368, -43.1416) (-15.0367, -43.1434) (-15.0354, -43.1613) (-15.0328, -43.1954) (-15.0289, -43.2458) (-15.0235, -43.3123) (-15.0166, -43.3934) (-15.0093, -43.4745) (-15.0017, -43.5556) (-14.9937, -43.6368) (-14.9853, -43.7181) (-14.9766, -43.7994) (-14.9676, -43.8807) (-14.9582, -43.9621) (-14.9485, -44.0436) (-14.9384, -44.125) (-14.928, -44.2065) (-14.9172, -44.2881) (-14.9061, -44.3697) (-14.8947, -44.4513) (-14.8829, -44.533) (-14.8709, -44.6147) (-14.8609, -44.6801) (-14.8533, -44.7291) (-14.8482, -44.7619) (-14.8456, -44.7782) knots 0.712736 0.712736 0.712736 0.712736 0.712736 0.712736 0.714286 0.728571 0.742857 0.757143 0.771429 0.785714 0.8 0.814286 0.828571 0.842857 0.857143 0.871429 0.885714 0.9 0.914286 0.928571 0.942857 0.957143 0.971429 0.985714 1 1 1 1 1 1
  arc A88 (-6.192, -46.7669) -> (-5.6329, -46.8375) centre (0, 0) ccw
  line L55 (-9.266, 28.1601) -> (-11.9496, 35.6966)
  spline S117 degree 3 poles (3.8356, 45.5258) (3.8568, 45.4628) (3.8901, 45.4046) (3.9771, 45.3043) (4.03, 45.2631) (4.1486, 45.2033) (4.2132, 45.1853) (4.3456, 45.175) (4.4122, 45.1829) (4.5386, 45.2236) (4.5972, 45.2562) (4.6943, 45.3381) (4.7333, 45.3852) (4.7631, 45.4381) knots 0 0 0 0 0.019923 0.019923 0.039846 0.039846 0.059769 0.059769 0.079691 0.079691 0.099614 0.099614 0.117812 0.117812 0.117812 0.117812
  spline S118 degree 3 poles (-39.5598, 22.8544) (-39.4939, 22.8468) (-39.427, 22.8522) (-39.2992, 22.8882) (-39.2394, 22.9185) (-39.1348, 23.0004) (-39.091, 23.0511) (-39.0253, 23.1666) (-39.0041, 23.2302) (-38.9871, 23.3619) (-38.9916, 23.4288) (-39.0245, 23.5515) (-39.0505, 23.6069) (-39.0856, 23.6563) knots 0 0 0 0 0.019923 0.019923 0.039846 0.039846 0.059769 0.059769 0.079691 0.079691 0.099614 0.099614 0.117812 0.117812 0.117812 0.117812
  spline S119 degree 5 poles (-47.0988, 2.6809) (-47.0845, 2.6724) (-47.056, 2.6556) (-47.0132, 2.6305) (-46.956, 2.5972) (-46.8845, 2.5559) (-46.8129, 2.5149) (-46.7412, 2.4742) (-46.6694, 2.4339) (-46.5976, 2.3938) (-46.5256, 2.3542) (-46.4536, 2.3148) (-46.3814, 2.2758) (-46.3092, 2.2371) (-46.2369, 2.1987) (-46.1645, 2.1607) (-46.092, 2.123) (-46.0195, 2.0857) (-45.9468, 2.0487) (-45.8741, 2.0121) (-45.8013, 1.9758) (-45.7414, 1.9463) (-45.6961, 1.9241) (-45.6653, 1.9092) (-45.6491, 1.9013) (-45.6475, 1.9006) knots -1 -1 -1 -1 -1 -1 -0.985714 -0.971429 -0.957143 -0.942857 -0.928571 -0.914286 -0.9 -0.885714 -0.871429 -0.857143 -0.842857 -0.828571 -0.814286 -0.8 -0.785714 -0.771429 -0.757143 -0.742857 -0.728571 -0.714286 -0.712736 -0.712736 -0.712736 -0.712736 -0.712736 -0.712736
  arc A89 (-14.3096, 44.9524) -> (-14.8456, 44.7782) centre (0, 0) ccw
  arc A90 (-11.4588, 45.7622) -> (-12.0047, 45.622) centre (0, 0) ccw
  arc A91 (20.3407, 42.5645) -> (19.8308, 42.8044) centre (0, 0) ccw
  spline S120 degree 5 poles (-39.5598, 22.8544) (-39.5616, 22.8546) (-39.5795, 22.8567) (-39.6135, 22.8606) (-39.6636, 22.8662) (-39.73, 22.8733) (-39.8109, 22.8817) (-39.892, 22.8898) (-39.9731, 22.8975) (-40.0544, 22.9048) (-40.1357, 22.9118) (-40.2172, 22.9185) (-40.2988, 22.9249) (-40.3805, 22.9309) (-40.4624, 22.9366) (-40.5443, 22.942) (-40.6263, 22.947) (-40.7084, 22.9517) (-40.7907, 22.9561) (-40.873, 22.9602) (-40.9554, 22.964) (-41.0379, 22.9674) (-41.104, 22.9699) (-41.1536, 22.9716) (-41.1867, 22.9727) (-41.2033, 22.9733) knots 0.712736 0.712736 0.712736 0.712736 0.712736 0.712736 0.714286 0.728571 0.742857 0.757143 0.771429 0.785714 0.8 0.814286 0.828571 0.842857 0.857143 0.871429 0.885714 0.9 0.914286 0.928571 0.942857 0.957143 0.971429 0.985714 1 1 1 1 1 1
  spline S121 degree 5 poles (25.2933, 38.0467) (25.2936, 38.0485) (25.2968, 38.0662) (25.3028, 38.0999) (25.3115, 38.1496) (25.3229, 38.2154) (25.3363, 38.2956) (25.3494, 38.376) (25.3622, 38.4565) (25.3747, 38.5371) (25.3868, 38.6179) (25.3986, 38.6988) (25.41, 38.7798) (25.4212, 38.861) (25.432, 38.9423) (25.4425, 39.0237) (25.4527, 39.1053) (25.4626, 39.1869) (25.4721, 39.2687) (25.4813, 39.3506) (25.4903, 39.4327) (25.4989, 39.5148) (25.5055, 39.5806) (25.5104, 39.63) (25.5135, 39.663) (25.5151, 39.6795) knots 0.712736 0.712736 0.712736 0.712736 0.712736 0.712736 0.714286 0.728571 0.742857 0.757143 0.771429 0.785714 0.8 0.814286 0.828571 0.842857 0.857143 0.871429 0.885714 0.9 0.914286 0.928571 0.942857 0.957143 0.971429 0.985714 1 1 1 1 1 1
  spline S122 degree 5 poles (-10.4204, 44.4828) (-10.4215, 44.4842) (-10.4322, 44.4987) (-10.4526, 44.5261) (-10.4829, 44.5665) (-10.5231, 44.6198) (-10.5724, 44.6845) (-10.622, 44.7491) (-10.6719, 44.8135) (-10.7222, 44.8778) (-10.7728, 44.9419) (-10.8237, 45.0059) (-10.8749, 45.0698) (-10.9265, 45.1334) (-10.9783, 45.197) (-11.0305, 45.2604) (-11.083, 45.3236) (-11.1357, 45.3867) (-11.1888, 45.4497) (-11.2422, 45.5125) (-11.2959, 45.5751) (-11.3499, 45.6376) (-11.3933, 45.6875) (-11.426, 45.7249) (-11.4479, 45.7497) (-11.4588, 45.7622) knots 0.712736 0.712736 0.712736 0.712736 0.712736 0.712736 0.714286 0.728571 0.742857 0.757143 0.771429 0.785714 0.8 0.814286 0.828571 0.842857 0.857143 0.871429 0.885714 0.9 0.914286 0.928571 0.942857 0.957143 0.971429 0.985714 1 1 1 1 1 1
  spline S123 degree 5 poles (-39.6795, -25.5151) (-39.663, -25.5135) (-39.63, -25.5104) (-39.5806, -25.5055) (-39.5148, -25.4989) (-39.4327, -25.4903) (-39.3506, -25.4813) (-39.2687, -25.4721) (-39.1869, -25.4626) (-39.1053, -25.4527) (-39.0237, -25.4425) (-38.9423, -25.432) (-38.861, -25.4212) (-38.7798, -25.41) (-38.6988, -25.3986) (-38.6179, -25.3868) (-38.5371, -25.3747) (-38.4565, -25.3622) (-38.376, -25.3494) (-38.2956, -25.3363) (-38.2154, -25.3229) (-38.1496, -25.3115) (-38.0999, -25.3028) (-38.0662, -25.2968) (-38.0485, -25.2936) (-38.0467, -25.2933) knots -1 -1 -1 -1 -1 -1 -0.985714 -0.971429 -0.957143 -0.942857 -0.928571 -0.914286 -0.9 -0.885714 -0.871429 -0.857143 -0.842857 -0.828571 -0.814286 -0.8 -0.785714 -0.771429 -0.757143 -0.742857 -0.728571 -0.714286 -0.712736 -0.712736 -0.712736 -0.712736 -0.712736 -0.712736
  spline S124 degree 3 poles (-13.1929, 43.7407) (-13.1501, 43.69) (-13.0977, 43.6482) (-12.9798, 43.5869) (-12.9155, 43.5681) (-12.7832, 43.5562) (-12.7165, 43.5632) (-12.5896, 43.6024) (-12.5306, 43.6342) (-12.4281, 43.7186) (-12.3855, 43.7704) (-12.3255, 43.8824) (-12.3066, 43.9406) (-12.2983, 44.0007) knots 0 0 0 0 0.019923 0.019923 0.039846 0.039846 0.059769 0.059769 0.079691 0.079691 0.099614 0.099614 0.117812 0.117812 0.117812 0.117812
  spline S125 degree 3 poles (-27.6324, -36.3835) (-27.6166, -36.319) (-27.6135, -36.252) (-27.6332, -36.1207) (-27.6558, -36.0575) (-27.7239, -35.9435) (-27.7688, -35.8937) (-27.8751, -35.8141) (-27.9355, -35.785) (-28.0641, -35.7517) (-28.131, -35.7477) (-28.2569, -35.7649) (-28.3151, -35.7838) (-28.3685, -35.8125) knots 0 0 0 0 0.019923 0.019923 0.039846 0.039846 0.059769 0.059769 0.079691 0.079691 0.099614 0.099614 0.117812 0.117812 0.117812 0.117812
  spline S126 degree 3 poles (-15.9134, 42.826) (-15.8674, 42.7781) (-15.8125, 42.7397) (-15.6911, 42.6859) (-15.6257, 42.6712) (-15.4929, 42.6676) (-15.4268, 42.6788) (-15.3026, 42.7258) (-15.2457, 42.7613) (-15.1487, 42.852) (-15.1095, 42.9064) (-15.0565, 43.0219) (-15.0413, 43.0811) (-15.0368, 43.1416) knots 0 0 0 0 0.019923 0.019923 0.039846 0.039846 0.059769 0.059769 0.079691 0.079691 0.099614 0.099614 0.117812 0.117812 0.117812 0.117812
  spline S127 degree 5 poles (-42.8044, 19.8308) (-42.7943, 19.8177) (-42.7739, 19.7916) (-42.7434, 19.7525) (-42.7025, 19.7005) (-42.6512, 19.6357) (-42.5997, 19.5713) (-42.5481, 19.5071) (-42.4962, 19.4431) (-42.4441, 19.3794) (-42.3918, 19.3161) (-42.3393, 19.2529) (-42.2866, 19.1901) (-42.2337, 19.1275) (-42.1806, 19.0652) (-42.1273, 19.0032) (-42.0738, 18.9415) (-42.02, 18.8801) (-41.9661, 18.819) (-41.912, 18.7582) (-41.8576, 18.6976) (-41.8128, 18.6481) (-41.7788, 18.6109) (-41.7557, 18.5856) (-41.7435, 18.5724) (-41.7423, 18.5711) knots -1 -1 -1 -1 -1 -1 -0.985714 -0.971429 -0.957143 -0.942857 -0.928571 -0.914286 -0.9 -0.885714 -0.871429 -0.857143 -0.842857 -0.828571 -0.814286 -0.8 -0.785714 -0.771429 -0.757143 -0.742857 -0.728571 -0.714286 -0.712736 -0.712736 -0.712736 -0.712736 -0.712736 -0.712736
  arc A92 (24.1926, 29.8428) -> (22.4832, 31.103) centre (0.7975, -0.1016) ccw
  arc A93 (-32.4983, -34.1956) -> (-32.0875, -34.5814) centre (0, 0) ccw
  spline S128 degree 5 poles (-4.7631, 45.4381) (-4.7639, 45.4396) (-4.7728, 45.4553) (-4.7896, 45.4851) (-4.8146, 45.5289) (-4.8478, 45.5869) (-4.8886, 45.6572) (-4.9297, 45.7275) (-4.9712, 45.7977) (-5.013, 45.8678) (-5.0551, 45.9377) (-5.0976, 46.0076) (-5.1404, 46.0774) (-5.1836, 46.147) (-5.2271, 46.2165) (-5.2709, 46.286) (-5.315, 46.3553) (-5.3595, 46.4245) (-5.4042, 46.4936) (-5.4493, 46.5626) (-5.4947, 46.6315) (-5.5405, 46.7003) (-5.5773, 46.7552) (-5.6051, 46.7964) (-5.6236, 46.8238) (-5.6329, 46.8375) knots 0.712736 0.712736 0.712736 0.712736 0.712736 0.712736 0.714286 0.728571 0.742857 0.757143 0.771429 0.785714 0.8 0.814286 0.828571 0.842857 0.857143 0.871429 0.885714 0.9 0.914286 0.928571 0.942857 0.957143 0.971429 0.985714 1 1 1 1 1 1
  arc A94 (-41.2033, 22.9733) -> (-41.4748, 22.4794) centre (0, 0) ccw
  arc A95 (-17.104, 43.9652) -> (-17.628, 43.7577) centre (0, 0) ccw
  spline S129 degree 5 poles (-31.9746, -32.6333) (-31.9752, -32.635) (-31.9816, -32.6518) (-31.9938, -32.6837) (-32.0117, -32.7309) (-32.0352, -32.7934) (-32.0634, -32.8697) (-32.0914, -32.9462) (-32.119, -33.0229) (-32.1463, -33.0998) (-32.1734, -33.1769) (-32.2001, -33.2541) (-32.2266, -33.3316) (-32.2527, -33.4092) (-32.2786, -33.4871) (-32.3042, -33.5651) (-32.3295, -33.6433) (-32.3544, -33.7216) (-32.3792, -33.8002) (-32.4036, -33.8789) (-32.4277, -33.9578) (-32.4516, -34.0369) (-32.4704, -34.1003) (-32.4844, -34.1479) (-32.4937, -34.1797) (-32.4983, -34.1956) knots 0.712736 0.712736 0.712736 0.712736 0.712736 0.712736 0.714286 0.728571 0.742857 0.757143 0.771429 0.785714 0.8 0.814286 0.828571 0.842857 0.857143 0.871429 0.885714 0.9 0.914286 0.928571 0.942857 0.957143 0.971429 0.985714 1 1 1 1 1 1
  spline S130 degree 3 poles (-29.8624, -34.5766) (-29.8426, -34.5132) (-29.8353, -34.4466) (-29.8467, -34.3143) (-29.8653, -34.2499) (-29.9261, -34.1318) (-29.9678, -34.0792) (-30.0689, -33.9931) (-30.1273, -33.9603) (-30.2536, -33.919) (-30.3201, -33.9108) (-30.4468, -33.9201) (-30.5061, -33.9353) (-30.5612, -33.9605) knots 0 0 0 0 0.019923 0.019923 0.039846 0.039846 0.059769 0.059769 0.079691 0.079691 0.099614 0.099614 0.117812 0.117812 0.117812 0.117812
  spline S131 degree 3 poles (-45.6768, 0.9694) (-45.6153, 0.9945) (-45.5593, 1.0314) (-45.4646, 1.1246) (-45.4268, 1.1799) (-45.3746, 1.3021) (-45.3607, 1.3676) (-45.3587, 1.5004) (-45.3707, 1.5664) (-45.4194, 1.69) (-45.4555, 1.7465) (-45.5434, 1.8382) (-45.5929, 1.8742) (-45.6475, 1.9006) knots 0 0 0 0 0.019923 0.019923 0.039846 0.039846 0.059769 0.059769 0.079691 0.079691 0.099614 0.099614 0.117812 0.117812 0.117812 0.117812
  spline S132 degree 5 poles (25.0393, 39.9814) (25.025, 39.973) (24.9965, 39.9561) (24.9539, 39.9307) (24.8972, 39.8967) (24.8265, 39.8539) (24.7561, 39.8109) (24.6859, 39.7677) (24.616, 39.7242) (24.5463, 39.6805) (24.4768, 39.6366) (24.4076, 39.5924) (24.3387, 39.548) (24.27, 39.5033) (24.2015, 39.4585) (24.1333, 39.4133) (24.0654, 39.368) (23.9978, 39.3224) (23.9304, 39.2765) (23.8632, 39.2305) (23.7964, 39.1841) (23.7416, 39.1459) (23.7004, 39.1168) (23.6724, 39.097) (23.6578, 39.0866) (23.6563, 39.0856) knots -1 -1 -1 -1 -1 -1 -0.985714 -0.971429 -0.957143 -0.942857 -0.928571 -0.914286 -0.9 -0.885714 -0.871429 -0.857143 -0.842857 -0.828571 -0.814286 -0.8 -0.785714 -0.771429 -0.757143 -0.742857 -0.728571 -0.714286 -0.712736 -0.712736 -0.712736 -0.712736 -0.712736 -0.712736
  arc A96 (-43.7577, 17.628) -> (-43.9652, 17.104) centre (0, 0) ccw
  arc A97 (-26.1662, -26.8777) -> (-24.6282, -28.3422) centre (0.7975, -0.1016) ccw
  arc A98 (27.9562, 37.9991) -> (27.5003, 38.3303) centre (0, 0) ccw
  spline S133 degree 5 poles (-46.8375, 5.6329) (-46.8238, 5.6236) (-46.7964, 5.6051) (-46.7552, 5.5773) (-46.7003, 5.5405) (-46.6315, 5.4947) (-46.5626, 5.4493) (-46.4936, 5.4042) (-46.4245, 5.3595) (-46.3553, 5.315) (-46.286, 5.2709) (-46.2165, 5.2271) (-46.147, 5.1836) (-46.0774, 5.1404) (-46.0076, 5.0976) (-45.9377, 5.0551) (-45.8678, 5.013) (-45.7977, 4.9712) (-45.7275, 4.9297) (-45.6572, 4.8886) (-45.5869, 4.8478) (-45.5289, 4.8146) (-45.4851, 4.7896) (-45.4553, 4.7728) (-45.4396, 4.7639) (-45.4381, 4.7631) knots -1 -1 -1 -1 -1 -1 -0.985714 -0.971429 -0.957143 -0.942857 -0.928571 -0.914286 -0.9 -0.885714 -0.871429 -0.857143 -0.842857 -0.828571 -0.814286 -0.8 -0.785714 -0.771429 -0.757143 -0.742857 -0.728571 -0.714286 -0.712736 -0.712736 -0.712736 -0.712736 -0.712736 -0.712736
  arc A99 (27.7612, 26.6745) -> (26.2232, 28.139) centre (0.7975, -0.1016) ccw
  arc A100 (25.5151, 39.6795) -> (25.0393, 39.9814) centre (0, 0) ccw